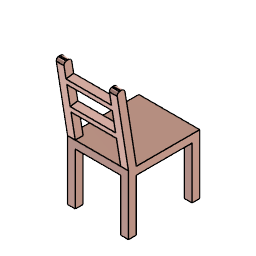
7- CREATE 3D MODEL FROM ORTHOGRAPHIC PROJECTION_ (Autodesk Fusion 360 design; units mm, degrees)
part number: 2026-03-11-19-21-16-020
Autodesk Fusion 360 part; units mm, degrees
sketch "Sketch1" plane through (0, 0, 0) normal (0, 1, 0) x (1, 0, 0)
  line L0 (0, 0) -> (-47, 0)
  line L1 (-47, 0) -> (-47, 6)
  line L2 (-47, 6) -> (0, 6)
  line L3 (0, 6) -> (0, 0)
  dimension "d1" = 47
  dimension "d2" = 6
  constraint horizontal L0
  constraint vertical L1
  constraint horizontal L2
  constraint vertical L3
  constraint coincident L0.start L3.end
  measures "d1" distance of L0.start L0.end
  measures "d2" distance of L0.start L2.end
extrude "Extrude1" add sketch "Sketch1" along normal blind 55
sketch "Sketch2" plane through (0, 0, -6) normal (0, 0, -1) x (1, 0, 0)
  line L0 (0, 0) -> (-47, 0)
  line L1 (-47, 0) -> (-47, -55)
  line L2 (-47, -55) -> (0, -55)
  line L3 (0, -55) -> (0, 0)
  line L4 (-47, 0) -> (-41, 0)
  line L5 (-41, 0) -> (-41, -6)
  line L6 (-41, -6) -> (-47, -6)
  line L7 (-47, -6) -> (-47, 0)
  line L8 (-6, 0) -> (0, 0)
  line L9 (-6, -6) -> (-6, 0)
  line L10 (0, -6) -> (-6, -6)
  line L11 (0, 0) -> (0, -6)
  line L12 (-47, -49) -> (-41, -49)
  line L13 (-47, -55) -> (-47, -49)
  line L14 (-41, -55) -> (-47, -55)
  line L15 (-41, -49) -> (-41, -55)
  line L16 (-6, -49) -> (0, -49)
  line L17 (-6, -55) -> (-6, -49)
  line L18 (0, -55) -> (-6, -55)
  line L19 (0, -49) -> (0, -55)
  dimension "d5" = 6
  dimension "d6" = 6
  dimension "d9" = 41
  dimension "d10" = -49
  constraint horizontal L4
  constraint vertical L5
  constraint horizontal L6
  constraint vertical L7
  constraint coincident L0.end L1.start
  measures "d5" distance of L5.end L6.end
  measures "d6" distance of L4.end L5.end
extrude "Extrude2" add sketch "Sketch2" along normal blind 40 contours L0 L3 L8 L9 L10 L11 | L0 L1 L4 L5 L6 L7 | L2 L3 L16 L17 L18 L19 | L1 L2 L12 L13 L14 L15
sketch "Sketch3" plane through (0, 0, 0) normal (1, 0, 0) x (0, 1, 0)
  line L0 (0, 0) -> (0, -46)
  line L1 (0, -46) -> (6, -46)
  line L2 (6, -46) -> (6, -6)
  line L3 (6, -6) -> (49, -6)
  line L4 (49, -6) -> (49, -46)
  line L5 (49, -46) -> (55, -46)
  line L6 (55, -46) -> (55, 0)
  line L7 (55, 0) -> (0, 0)
  line L8 (0, 0) -> (-9, 56)
  line L9 (-9, 56) -> (-3.076, 56.9521)
  line L10 (-3.076, 56.9521) -> (6.077, 0)
  line L11 (0.1627, 0) -> (6.077, 0)
  dimension "d14" = 56
  dimension "d15" = 6
  dimension "d45" = 64
  constraint coincident L0.start L7.end
  constraint perpendicular L8 L9
  constraint coincident L7 L10.end
  constraint perpendicular L9 L10
  constraint coincident L7 L11.start
  measures "d14" vertical distance of L0.start L8.end
  measures "d15" distance of L8.end L9.end
  measures "d45" horizontal distance of L6.end L8.end
sketch "Sketch4" plane through (0, 0, 0) normal (1, 0, 0) x (0, 1, 0)
extrude "Extrude3" add sketch "Sketch3" against normal blind 6 contours L7 L8 L9 L10 L11
fillet "Fillet1" radius 3 1 edges at (-3, -3.076, 56.9521)
fillet "Fillet2" radius 2 1 edges at (-3, -9, 56)
pattern_linear "R-Pattern1" count 2 spacing 41 along (-1, 0, 0) of "Extrude3"
fillet "Fillet3" radius 3 1 edges at (-44, -3.076, 56.9521)
fillet "Fillet4" radius 2 1 edges at (-44, -9, 56)
sketch "Sketch5" plane through (-41, 0, 0) normal (1, 0, 0) x (0, 1, 0)
  arc A0 (-7.0253, 56.3174) -> (-8.6826, 54.0253) centre (-6.708, 54.3427) ccw
  line L0 (-8.6826, 54.0253) -> (0, 0)
  line L1 (0, 0) -> (6.077, 0)
  line L2 (6.077, 0) -> (-2.6, 53.9901)
  arc A1 (-2.6, 53.9901) -> (-6.038, 56.476) centre (-5.562, 53.514) ccw
  line L3 (-6.038, 56.476) -> (-7.0253, 56.3174)
  line L4 (-7.1224, 44.3174) -> (-1.1985, 45.2694)
  line L5 (-1.1985, 45.2694) -> (-0.5556, 41.2694)
  line L6 (-0.5556, 41.2694) -> (-6.4796, 40.3174)
  line L7 (-7.1224, 44.3174) -> (-6.4796, 40.3174)
  line L8 (-3.9081, 24.3174) -> (2.0158, 25.2694)
  line L9 (2.0158, 25.2694) -> (2.6587, 21.2694)
  line L10 (2.6587, 21.2694) -> (-3.2653, 20.3174)
  line L11 (-3.9081, 24.3174) -> (-3.2653, 20.3174)
  dimension "d40" = 12
  dimension "d41" = 4
  dimension "d42" = 16
  dimension "d43" = 4
  constraint coincident L0 L4.start
  constraint perpendicular L0 L4
  constraint coincident L2 L4.end
  constraint coincident L2 L5.end
  constraint coincident L0 L6.end
  constraint perpendicular L0 L6
  constraint coincident L0 L8.start
  constraint perpendicular L0 L8
  constraint coincident L2 L8.end
  constraint coincident L2 L9.end
  constraint coincident L0 L10.end
  constraint perpendicular L0 L10
  measures "d40" vertical distance of A0.start L4.start
  measures "d41" vertical distance of L4.start L6.end
  measures "d42" vertical distance of L6.end L8.start
  measures "d43" vertical distance of L8.start L10.end
extrude "Extrude4" add sketch "Sketch5" along normal blind 35 contours L0 L2 L4 L5 L6 L7 | L0 L2 L8 L9 L10 L11
